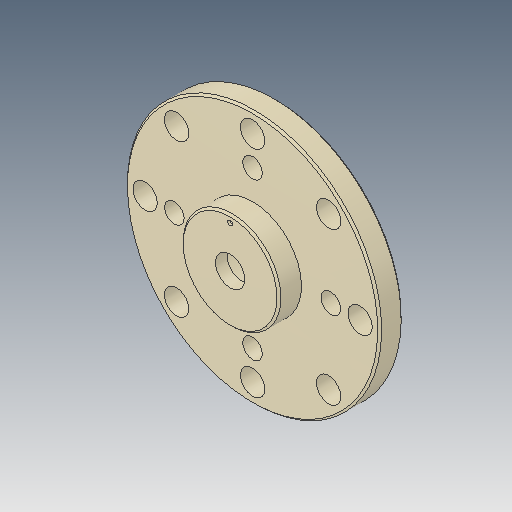
# Autodesk Inventor part: XM540_HORN
Saved by Autodesk Inventor 2019.4 (Build 234330000, 330)
## iProperties
Created: 2019-10-21
Part Number: XM540_HORN
Material: 一般
Document SubType Name: Modeling
Designer: y6tada
Density: 1 g/cm^3
Appearance: 淡いベージュ
Mass: 1.19114 g
Surface Area: 15.4404 cm^2
Volume: 1.19114 cm^3
Author: y6tada
Autodesk Inventor part; units mm, degrees
ref_plane "YZ Plane" through (0, 0, 0) normal (1, 0, 0) x (0, 1, 0)
ref_plane "XZ Plane" through (0, 0, 0) normal (0, 1, 0) x (-1, 0, 0)
ref_plane "XY Plane" through (0, 0, 0) normal (0, 0, 1) x (1, 0, 0)
sketch "スケッチ1" plane through (0, 0, 0) normal (1, 0, 0) x (0, 1, 0)
  line L0 (0, 0) -> (0, 18.1138) construction
  line L1 (1.5, 4.9) -> (1.5, 3.7)
  line L2 (1.5, 3.7) -> (4, 3.7)
  line L3 (4, 3.7) -> (4, -0.4)
  line L4 (4, -0.4) -> (4.95, -0.4)
  line L5 (4.95, -0.4) -> (4.95, 0)
  line L6 (4.95, 0) -> (9, 0)
  line L7 (9, 0) -> (9, 0.2)
  line L8 (9, 0.2) -> (13, 0.2)
  line L9 (13, 0.2) -> (13, 2.6)
  line L10 (13, 2.6) -> (5, 2.6)
  line L11 (5, 2.6) -> (5, 4.9)
  line L12 (5, 4.9) -> (1.5, 4.9)
  dimension "d0" = 9.9
  dimension "d1" = 10
  dimension "d2" = 5.3
  dimension "d3" = 4.1
  dimension "d4" = 3
  dimension "d5" = 2.6
  dimension "d6" = 2.4
  dimension "d7" = 26
  dimension "d8" = 18
  dimension "d9" = 8
  dimension "d10" = 2.3
  dimension "d43" = 3.7
  constraints: 26 end point, 11 perpendicular, 2 vertical, 1 point on line
  measures "d0" diameter of L5 L0
  measures "d1" diameter of L11 L0
  measures "d2" distance between parallel lines of L4 L12
  measures "d3" distance of L2.end L3.end
  measures "d4" diameter of L1 L0
  measures "d5" distance between parallel lines of L6 L10
  measures "d6" distance of L8.end L9.end
  measures "d7" diameter of L9 L0
  measures "d8" diameter of L7 L0
  measures "d9" diameter of L3 L0
  measures "d10" distance between parallel lines of L10 L12
  measures "d43" distance between parallel lines of L2 L6
revolve "回転1" add sketch "スケッチ1" angle 360 about axis through (0, 0, 0) along (0, 0, 1)
sketch "スケッチ2" plane through (0, 0, 2.6) normal (0, 0, 1) x (1, 0, 0)
  circle A0 centre (0, 0) radius 8 construction
  line L0 (0, 0) -> (0, 8) construction
  point P0 (-8, 0)
  point P1 (-8, 0)
  point P2 (0, -8)
  point P3 (0, -8)
  point P4 (8, 0)
  point P5 (8, 0)
  dimension "d12" = 16
  dimension "d15" = 360
  constraints: 5 coincident, 2 end point, 1 vertical, 1 vertical alignment, 11 other
hole "穴1" at (0, 8, 2.6) at (-8, 0, 2.6) at (0, -8, 2.6) at (8, 0, 2.6) direction (0, 0, -1) diameter 2 end through all
sketch "スケッチ3" plane through (0, 0, 2.6) normal (0, 0, 1) x (1, 0, 0)
  line L0 (0, 0) -> (0, 11) construction
  point P0 (-7.7782, 7.7782)
  point P1 (-11, 0)
  point P2 (-7.7782, -7.7782)
  point P3 (0, -11)
  point P4 (7.7782, -7.7782)
  point P5 (11, 0)
  point P6 (7.7782, 7.7782)
  dimension "d25" = 11
  dimension "d28" = 360
  constraints: 2 end point, 1 coincident, 1 vertical, 9 other
  measures "d25" distance of L0.start L0.end
hole "穴2" at (0, 11, 2.6) at (-7.7782, 7.7782, 2.6) at (-11, 0, 2.6) at (-7.7782, -7.7782, 2.6) at (0, -11, 2.6) at (7.7782, -7.7782, 2.6) at (11, 0, 2.6) at (7.7782, 7.7782, 2.6) direction (0, 0, -1) diameter 2.5 end through all
chamfer "面取り1" distance 0.2 angle 45 3 edges at (0, -13, 2.6) (0, -13, 0.2) (0, -5, 4.9)
sketch "スケッチ4" plane through (0, 0, 4.9) normal (0, 0, 1) x (1, 0, 0)
  line L0 (0, 0) -> (0, 4.25) construction
  dimension "d44" = 4.25
  constraints: 2 end point, 1 coincident, 1 vertical
  measures "d44" distance of L0.start L0.end
hole "穴3" at (0, 4.25, 4.9) direction (0, 0, -1) diameter 0.5 depth 0.25 tip angle 118
